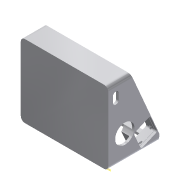
# Autodesk Inventor part: 03_OpenOxygen_Box
Saved by Autodesk Inventor 2019.4 (Build 234330000, 330)
## iProperties
Created: 2021-06-03
Part Number: 03_OpenOxygen_Box
Material: Generic
Document SubType Name: Modeling
Designer: diederichbenedict
Density: 1 g/cm^3
Appearance: Snow
Author: diederichbenedict
Autodesk Inventor part; units mm, degrees
(part 1 of 2)
ref_plane "YZ Plane" through (0, 0, 0) normal (1, 0, 0) x (0, 1, 0)
ref_plane "XZ Plane" through (0, 0, 0) normal (0, 1, 0) x (-1, 0, 0)
ref_plane "Work Plane1" through (0, 0, 0) normal (0, 0, 1) x (1, 0, 0)
sketch "Sketch1" plane through (0, 0, 0) normal (0, 0, 1) x (1, 0, 0)
  line L0 (30.9254, 0.1) -> (30.9254, 0) projected
  line L1 (30.9254, 0) -> (32.2546, 0) projected
  line L2 (32.2546, 0) -> (32.2546, 0.1) projected
  line L3 (32.2546, 0.1) -> (33.4654, 0.1) projected
  line L4 (33.4654, 0.1) -> (33.4654, 0) projected
  line L5 (33.4654, 0) -> (34.7946, 0) projected
  line L6 (34.7946, 0) -> (34.7946, 0.1) projected
  line L7 (34.7946, 0.1) -> (36.0054, 0.1) projected
  line L8 (36.0054, 0.1) -> (36.0054, 0) projected
  line L9 (36.0054, 0) -> (37.3346, 0) projected
  line L10 (37.3346, 0) -> (37.3346, 0.1) projected
  line L11 (37.3346, 0.1) -> (38.5454, 0.1) projected
  line L12 (38.5454, 0.1) -> (38.5454, 0) projected
  line L13 (38.5454, 0) -> (39.8746, 0) projected
  line L14 (39.8746, 0) -> (39.8746, 0.1) projected
  line L15 (39.8746, 0.1) -> (41.0854, 0.1) projected
  line L16 (41.0854, 0.1) -> (41.0854, 0) projected
  line L17 (41.0854, 0) -> (42.4146, 0) projected
  line L18 (42.4146, 0) -> (42.4146, 0.1) projected
  line L19 (42.4146, 0.1) -> (43.6254, 0.1) projected
  line L20 (43.6254, 0.1) -> (43.6254, 0) projected
  line L21 (43.6254, 0) -> (44.9546, 0) projected
  line L22 (44.9546, 0) -> (44.9546, 0.1) projected
  line L23 (44.9546, 0.1) -> (46.1654, 0.1) projected
  line L24 (46.1654, 0.1) -> (46.1654, 0) projected
  line L25 (46.1654, 0) -> (47.4946, 0) projected
  line L26 (47.4946, 0) -> (47.4946, 0.1) projected
  line L27 (47.4946, 0.1) -> (48.7054, 0.1) projected
  line L28 (48.7054, 0.1) -> (48.7054, 0) projected
  line L29 (48.7054, 0) -> (98, 0) projected
  line L30 (98, 0) -> (98, 1.6) projected
  line L31 (0, 1.6) -> (98, 1.6) projected
  line L32 (0, 0) -> (0, 1.6) projected
  line L33 (0, 0) -> (9.3946, 0) projected
  line L34 (9.3946, 0) -> (9.3946, 0.1) projected
  line L35 (9.3946, 0.1) -> (10.6054, 0.1) projected
  line L36 (10.6054, 0.1) -> (10.6054, 0) projected
  line L37 (10.6054, 0) -> (11.9346, 0) projected
  line L38 (11.9346, 0) -> (11.9346, 0.1) projected
  line L39 (11.9346, 0.1) -> (13.1454, 0.1) projected
  line L40 (13.1454, 0.1) -> (13.1454, 0) projected
  line L41 (13.1454, 0) -> (14.4746, 0) projected
  line L42 (14.4746, 0) -> (14.4746, 0.1) projected
  line L43 (14.4746, 0.1) -> (15.6854, 0.1) projected
  line L44 (15.6854, 0.1) -> (15.6854, 0) projected
  line L45 (15.6854, 0) -> (17.0146, 0) projected
  line L46 (17.0146, 0) -> (17.0146, 0.1) projected
  line L47 (17.0146, 0.1) -> (18.2254, 0.1) projected
  line L48 (18.2254, 0.1) -> (18.2254, 0) projected
  line L49 (18.2254, 0) -> (19.5546, 0) projected
  line L50 (19.5546, 0) -> (19.5546, 0.1) projected
  line L51 (19.5546, 0.1) -> (20.7654, 0.1) projected
  line L52 (20.7654, 0.1) -> (20.7654, 0) projected
  line L53 (20.7654, 0) -> (22.0946, 0) projected
  line L54 (22.0946, 0) -> (22.0946, 0.1) projected
  line L55 (22.0946, 0.1) -> (23.3054, 0.1) projected
  line L56 (23.3054, 0.1) -> (23.3054, 0) projected
  line L57 (23.3054, 0) -> (24.6346, 0) projected
  line L58 (24.6346, 0) -> (24.6346, 0.1) projected
  line L59 (24.6346, 0.1) -> (25.8454, 0.1) projected
  line L60 (25.8454, 0.1) -> (25.8454, 0) projected
  line L61 (25.8454, 0) -> (27.1746, 0) projected
  line L62 (27.1746, 0) -> (27.1746, 0.1) projected
  line L63 (27.1746, 0.1) -> (28.3854, 0.1) projected
  line L64 (28.3854, 0.1) -> (28.3854, 0) projected
  line L65 (28.3854, 0) -> (29.7146, 0) projected
  line L66 (29.7146, 0) -> (29.7146, 0.1) projected
  line L67 (29.7146, 0.1) -> (30.9254, 0.1) projected
  line L68 (63.1351, 91.3523) -> (63.1351, 51.3523) projected
  line L69 (49.1351, 91.3523) -> (63.1351, 91.3523) projected
  line L70 (49.1351, 51.3523) -> (49.1351, 91.3523) projected
  line L71 (63.1351, 51.3523) -> (49.1351, 51.3523) projected
  line L72 (0, 1.6) -> (98, 1.6)
  line L73 (103, 6.6) -> (103, 86.6)
  line L74 (98, 91.6) -> (0, 91.6)
  line L75 (-5, 86.6) -> (-5, 6.6)
  arc A0 (98, 1.6) -> (103, 6.6) centre (98, 6.6) ccw
  arc A1 (103, 86.6) -> (98, 91.6) centre (98, 86.6) ccw
  arc A2 (0, 91.6) -> (-5, 86.6) centre (0, 86.6) ccw
  arc A3 (-5, 6.6) -> (0, 1.6) centre (0, 6.6) ccw
  point P0 (-5, 1.6)
  point P1 (103, 91.6)
  point P2 (103, 1.6)
  point P3 (-5, 91.6)
  dimension "d1" = 5
  dimension "d2" = 5
  dimension "d3" = 90
  dimension "d6" = 5
  constraints: 9 point on line, 8 end point, 8 point on circle, 8 tangent, 4 centre point, 3 equal radius, 2 parallel, 1 horizontal, 1 perpendicular
  measures "d1" distance between parallel lines of L32 L75
  measures "d2" distance between parallel lines of L30 L73
  measures "d3" distance between parallel lines of L72 L74
  measures "d6" radius of A0
extrude "Extrusion1" add sketch "Sketch1" along normal blind 3 contours L31 A3 L75 A2 L74 A1 L73 A0 | L68 L71 L70 L69
sketch "Sketch2" plane through (0, 0, 0) normal (0, 0, -1) x (-1, 0, 0)
  arc A0 (0, 1.6) -> (5, 6.6) centre (0, 6.6) ccw projected
  line L0 (5, 6.6) -> (5, 86.6) projected
  arc A1 (5, 86.6) -> (0, 91.6) centre (0, 86.6) ccw projected
  line L1 (0, 91.6) -> (-98, 91.6) projected
  arc A2 (-98, 91.6) -> (-103, 86.6) centre (-98, 86.6) ccw projected
  line L2 (-103, 86.6) -> (-103, 6.6) projected
  arc A3 (-103, 6.6) -> (-98, 1.6) centre (-98, 6.6) ccw projected
  line L3 (-98, 1.6) -> (0, 1.6) projected
  line L4 (-100, 6.6) -> (-100, 86.6)
  arc A4 (-98, 88.6) -> (-100, 86.6) centre (-98, 86.6) ccw
  line L5 (-98, 88.6) -> (0, 88.6)
  arc A5 (2, 86.6) -> (0, 88.6) centre (0, 86.6) ccw
  line L6 (2, 86.6) -> (2, 6.6)
  arc A6 (0, 4.6) -> (2, 6.6) centre (0, 6.6) ccw
  line L7 (0, 4.6) -> (-98, 4.6)
  arc A7 (-100, 6.6) -> (-98, 4.6) centre (-98, 6.6) ccw
  point P0 (0, 0)
  dimension "d7" = 3
  constraints: 8 end point, 8 point on circle, 4 centre point, 7 other
  measures "d7" distance between parallel lines of L2 L4
ref_plane "Work Plane2" through (0, 0, -60) normal (0, 0, -1) x (0, 1, 0)
extrude "Extrusion2" add sketch "Sketch2" along normal up to surface (60 mm away)
sketch "Sketch3" plane through (-5, 6.6, 3) normal (-1, 0, 0) x (0, 0, 1)
  line L0 (0, 0) -> (-63, 0) projected
  line L1 (0, 80) -> (0, 0) projected
  line L2 (0, 80) -> (-63, 80) projected
  line L3 (-63, 80) -> (-63, 0) projected
  line L4 (-63, 4.0286) -> (-27.0673, 87.1327)
  line L5 (-27.0673, 87.1327) -> (-72.7137, 86.3795)
  line L6 (-72.7137, 86.3795) -> (-69.4498, 6.2882)
  line L7 (-69.4498, 6.2882) -> (-63, 4.0286)
  point P0 (-3, -6.6)
  constraints: 8 end point, 1 point on line
extrude "Extrusion3" cut sketch "Sketch3" against normal through all contours L7 L6 L5 L4 L2 L3 | L3 L2 L4
sketch "Sketch4" plane through (-5, 6.6, 3) normal (-1, 0, 0) x (0, 0, 1)
  circle A0 centre (-20.557, 24.8509) radius 11.8979 projected
  point P0 (-3, -6.6)
extrude "Extrusion4" cut sketch "Sketch4" against normal through all
sketch "Sketch5" plane through (0, 1.6, 3) normal (0, -1, 0) x (1, 0, 0)
  circle A0 centre (95.5, -5.5) radius 1.5 projected
  circle A1 centre (95.5, -60.5) radius 1.5 projected
  circle A2 centre (2.5, -60.5) radius 1.5 projected
  circle A3 centre (2.5, -5.5) radius 1.5 projected
  line L0 (8.1, -22.25) -> (8.1, -4.25) construction
  line L1 (8.1, -4.25) -> (49.6, -4.25) construction
  line L2 (49.6, -4.25) -> (49.6, -22.25) construction
  line L3 (49.6, -22.25) -> (8.1, -22.25) construction
  circle A4 centre (43.02, -5.5) radius 0.75 construction
  circle A5 centre (40.48, -5.5) radius 0.75 construction
  circle A6 centre (37.94, -5.5) radius 0.75 construction
  circle A7 centre (35.4, -5.5) radius 0.75 construction
  circle A8 centre (32.86, -5.5) radius 0.75 construction
  circle A9 centre (30.32, -5.5) radius 0.75 construction
  circle A10 centre (27.78, -5.5) radius 0.75 construction
  circle A11 centre (25.24, -5.5) radius 0.75 construction
  circle A12 centre (22.7, -5.5) radius 0.75 construction
  circle A13 centre (20.16, -5.5) radius 0.75 construction
  circle A14 centre (17.62, -5.5) radius 0.75 construction
  circle A15 centre (15.08, -5.5) radius 0.75 construction
  circle A16 centre (12.54, -5.5) radius 0.75 construction
  circle A17 centre (10, -5.5) radius 0.75 construction
  line L4 (21.6, -15.05) -> (14.6, -15.05) construction
  line L5 (21.6, -8.05) -> (21.6, -15.05) construction
  line L6 (14.6, -8.05) -> (21.6, -8.05) construction
  line L7 (14.6, -15.05) -> (14.6, -8.05) construction
  line L8 (20.85, -20.75) -> (19.85, -20.75) construction
  line L9 (20.85, -19.25) -> (20.85, -20.75) construction
  line L10 (19.85, -19.25) -> (20.85, -19.25) construction
  line L11 (19.85, -20.75) -> (19.85, -19.25) construction
  line L12 (20.85, -18.75) -> (19.85, -18.75) construction
  line L13 (20.85, -17.25) -> (20.85, -18.75) construction
  line L14 (19.85, -17.25) -> (20.85, -17.25) construction
  line L15 (19.85, -18.75) -> (19.85, -17.25) construction
  line L16 (17.85, -20.75) -> (17.85, -19.25) construction
  line L17 (18.85, -20.75) -> (17.85, -20.75) construction
  line L18 (18.85, -19.25) -> (18.85, -20.75) construction
  line L19 (17.85, -19.25) -> (18.85, -19.25) construction
  line L20 (17.85, -18.75) -> (17.85, -17.25) construction
  line L21 (18.85, -18.75) -> (17.85, -18.75) construction
  line L22 (18.85, -17.25) -> (18.85, -18.75) construction
  line L23 (17.85, -17.25) -> (18.85, -17.25) construction
  line L24 (15.85, -20.75) -> (15.85, -19.25) construction
  line L25 (16.85, -20.75) -> (15.85, -20.75) construction
  line L26 (16.85, -19.25) -> (16.85, -20.75) construction
  line L27 (15.85, -19.25) -> (16.85, -19.25) construction
  line L28 (15.85, -18.75) -> (15.85, -17.25) construction
  line L29 (16.85, -18.75) -> (15.85, -18.75) construction
  line L30 (16.85, -17.25) -> (16.85, -18.75) construction
  line L31 (15.85, -17.25) -> (16.85, -17.25) construction
  line L32 (36.6, -19.725) -> (37.6, -19.725) construction
  line L33 (36.6, -19.75) -> (36.6, -19.725) construction
  line L34 (36.1, -19.75) -> (36.6, -19.75) construction
  line L35 (36.1, -21) -> (36.1, -19.75) construction
  line L36 (36.6, -21) -> (36.1, -21) construction
  line L37 (36.6, -21.025) -> (36.6, -21) construction
  line L38 (37.6, -21.025) -> (36.6, -21.025) construction
  line L39 (37.6, -21) -> (37.6, -21.025) construction
  line L40 (38.1, -21) -> (37.6, -21) construction
  line L41 (38.1, -19.75) -> (38.1, -21) construction
  line L42 (37.6, -19.75) -> (38.1, -19.75) construction
  line L43 (37.6, -19.725) -> (37.6, -19.75) construction
  line L44 (31.6, -21) -> (31.1, -21) construction
  line L45 (31.6, -21.025) -> (31.6, -21) construction
  line L46 (32.6, -21.025) -> (31.6, -21.025) construction
  line L47 (32.6, -21) -> (32.6, -21.025) construction
  line L48 (33.1, -21) -> (32.6, -21) construction
  line L49 (33.1, -19.75) -> (33.1, -21) construction
  line L50 (32.6, -19.75) -> (33.1, -19.75) construction
  line L51 (32.6, -19.725) -> (32.6, -19.75) construction
  line L52 (31.6, -19.725) -> (32.6, -19.725) construction
  line L53 (31.6, -19.75) -> (31.6, -19.725) construction
  line L54 (31.1, -19.75) -> (31.6, -19.75) construction
  line L55 (31.1, -21) -> (31.1, -19.75) construction
  line L56 (26.6, -21) -> (26.1, -21) construction
  line L57 (26.6, -21.025) -> (26.6, -21) construction
  line L58 (27.6, -21.025) -> (26.6, -21.025) construction
  line L59 (27.6, -21) -> (27.6, -21.025) construction
  line L60 (28.1, -21) -> (27.6, -21) construction
  line L61 (28.1, -19.75) -> (28.1, -21) construction
  line L62 (27.6, -19.75) -> (28.1, -19.75) construction
  line L63 (27.6, -19.725) -> (27.6, -19.75) construction
  line L64 (26.6, -19.725) -> (27.6, -19.725) construction
  line L65 (26.6, -19.75) -> (26.6, -19.725) construction
  line L66 (26.1, -19.75) -> (26.6, -19.75) construction
  line L67 (26.1, -21) -> (26.1, -19.75) construction
  line L68 (45.1607, -15.4113) -> (45.1607, -14.9113) construction
  line L69 (45.1357, -15.4113) -> (45.1607, -15.4113) construction
  line L70 (45.1357, -16.4113) -> (45.1357, -15.4113) construction
  line L71 (45.1607, -16.4113) -> (45.1357, -16.4113) construction
  line L72 (45.1607, -16.9113) -> (45.1607, -16.4113) construction
  line L73 (46.4107, -16.9113) -> (45.1607, -16.9113) construction
  line L74 (46.4107, -16.4113) -> (46.4107, -16.9113) construction
  line L75 (46.4357, -16.4113) -> (46.4107, -16.4113) construction
  line L76 (46.4357, -15.4113) -> (46.4357, -16.4113) construction
  line L77 (46.4107, -15.4113) -> (46.4357, -15.4113) construction
  line L78 (46.4107, -14.9113) -> (46.4107, -15.4113) construction
  line L79 (45.1607, -14.9113) -> (46.4107, -14.9113) construction
  line L80 (42.6357, -16.4113) -> (42.6357, -15.4113) construction
  line L81 (42.6607, -16.4113) -> (42.6357, -16.4113) construction
  line L82 (42.6607, -16.9113) -> (42.6607, -16.4113) construction
  line L83 (43.9107, -16.9113) -> (42.6607, -16.9113) construction
  line L84 (43.9107, -16.4113) -> (43.9107, -16.9113) construction
  line L85 (43.9357, -16.4113) -> (43.9107, -16.4113) construction
  line L86 (43.9357, -15.4113) -> (43.9357, -16.4113) construction
  line L87 (43.9107, -15.4113) -> (43.9357, -15.4113) construction
  line L88 (43.9107, -14.9113) -> (43.9107, -15.4113) construction
  line L89 (42.6607, -14.9113) -> (43.9107, -14.9113) construction
  line L90 (42.6607, -15.4113) -> (42.6607, -14.9113) construction
  line L91 (42.6357, -15.4113) -> (42.6607, -15.4113) construction
  line L92 (40.1357, -16.4113) -> (40.1357, -15.4113) construction
  line L93 (40.1607, -16.4113) -> (40.1357, -16.4113) construction
  line L94 (40.1607, -16.9113) -> (40.1607, -16.4113) construction
  line L95 (41.4107, -16.9113) -> (40.1607, -16.9113) construction
  line L96 (41.4107, -16.4113) -> (41.4107, -16.9113) construction
  line L97 (41.4357, -16.4113) -> (41.4107, -16.4113) construction
  line L98 (41.4357, -15.4113) -> (41.4357, -16.4113) construction
  line L99 (41.4107, -15.4113) -> (41.4357, -15.4113) construction
  line L100 (41.4107, -14.9113) -> (41.4107, -15.4113) construction
  line L101 (40.1607, -14.9113) -> (41.4107, -14.9113) construction
  line L102 (40.1607, -15.4113) -> (40.1607, -14.9113) construction
  line L103 (40.1357, -15.4113) -> (40.1607, -15.4113) construction
  line L104 (37.6357, -16.4113) -> (37.6357, -15.4113) construction
  line L105 (37.6607, -16.4113) -> (37.6357, -16.4113) construction
  line L106 (37.6607, -16.9113) -> (37.6607, -16.4113) construction
  line L107 (38.9107, -16.9113) -> (37.6607, -16.9113) construction
  line L108 (38.9107, -16.4113) -> (38.9107, -16.9113) construction
  line L109 (38.9357, -16.4113) -> (38.9107, -16.4113) construction
  line L110 (38.9357, -15.4113) -> (38.9357, -16.4113) construction
  line L111 (38.9107, -15.4113) -> (38.9357, -15.4113) construction
  line L112 (38.9107, -14.9113) -> (38.9107, -15.4113) construction
  line L113 (37.6607, -14.9113) -> (38.9107, -14.9113) construction
  line L114 (37.6607, -15.4113) -> (37.6607, -14.9113) construction
  line L115 (37.6357, -15.4113) -> (37.6607, -15.4113) construction
  line L116 (40.1607, -10.9113) -> (40.1607, -10.4113) construction
  line L117 (40.1357, -10.9113) -> (40.1607, -10.9113) construction
  line L118 (40.1357, -11.9113) -> (40.1357, -10.9113) construction
  line L119 (40.1607, -11.9113) -> (40.1357, -11.9113) construction
  line L120 (40.1607, -12.4113) -> (40.1607, -11.9113) construction
  line L121 (41.4107, -12.4113) -> (40.1607, -12.4113) construction
  line L122 (41.4107, -11.9113) -> (41.4107, -12.4113) construction
  line L123 (41.4357, -11.9113) -> (41.4107, -11.9113) construction
  line L124 (41.4357, -10.9113) -> (41.4357, -11.9113) construction
  line L125 (41.4107, -10.9113) -> (41.4357, -10.9113) construction
  line L126 (41.4107, -10.4113) -> (41.4107, -10.9113) construction
  line L127 (40.1607, -10.4113) -> (41.4107, -10.4113) construction
  line L128 (37.6357, -11.9113) -> (37.6357, -10.9113) construction
  line L129 (37.6607, -11.9113) -> (37.6357, -11.9113) construction
  line L130 (37.6607, -12.4113) -> (37.6607, -11.9113) construction
  line L131 (38.9107, -12.4113) -> (37.6607, -12.4113) construction
  line L132 (38.9107, -11.9113) -> (38.9107, -12.4113) construction
  line L133 (38.9357, -11.9113) -> (38.9107, -11.9113) construction
  line L134 (38.9357, -10.9113) -> (38.9357, -11.9113) construction
  line L135 (38.9107, -10.9113) -> (38.9357, -10.9113) construction
  line L136 (38.9107, -10.4113) -> (38.9107, -10.9113) construction
  line L137 (37.6607, -10.4113) -> (38.9107, -10.4113) construction
  line L138 (37.6607, -10.9113) -> (37.6607, -10.4113) construction
  line L139 (37.6357, -10.9113) -> (37.6607, -10.9113) construction
  line L140 (43.4, -11.75) -> (43.2, -11.75) construction
  line L141 (43.4, -12.45) -> (43.4, -11.75) construction
  line L142 (43.9, -12.45) -> (43.4, -12.45) construction
  line L143 (43.9, -11.75) -> (43.9, -12.45) construction
  line L144 (45.2, -11.75) -> (43.9, -11.75) construction
  line L145 (45.2, -12.45) -> (45.2, -11.75) construction
  line L146 (45.7, -12.45) -> (45.2, -12.45) construction
  line L147 (45.7, -11.75) -> (45.7, -12.45) construction
  line L148 (45.9, -11.75) -> (45.7, -11.75) construction
  line L149 (45.9, -10.25) -> (45.9, -11.75) construction
  line L150 (44.8, -10.25) -> (45.9, -10.25) construction
  line L151 (44.8, -9.55) -> (44.8, -10.25) construction
  line L152 (44.3, -9.55) -> (44.8, -9.55) construction
  line L153 (44.3, -10.25) -> (44.3, -9.55) construction
  line L154 (43.2, -10.25) -> (44.3, -10.25) construction
  line L155 (43.2, -11.75) -> (43.2, -10.25) construction
  line L156 (11.6965, -17.6363) -> (11.6965, -16.6863) construction
  line L157 (11.6965, -16.6863) -> (11.6112, -16.6863) construction
  line L158 (11.6112, -16.6863) -> (11.6112, -17.5389) construction
  line L159 (11.6112, -17.5389) -> (11.2458, -17.5389) construction
  line L160 (11.2458, -17.5389) -> (11.2458, -17.6363) construction
  line L161 (11.2458, -17.6363) -> (11.6965, -17.6363) construction
  spline S0 degree 3 poles (12.3058, -16.662) (12.2949, -16.6621) (12.2733, -16.6624) (12.2413, -16.6649) (12.2102, -16.6691) (12.1799, -16.6748) (12.1503, -16.6819) (12.1216, -16.6912) (12.0936, -16.7018) (12.0665, -16.714) (12.0405, -16.7277) (12.0155, -16.7427) (11.9918, -16.7591) (11.9691, -16.7767) (11.9479, -16.7958) (11.9276, -16.8159) (11.9088, -16.8377) (11.8972, -16.853) (11.8913, -16.8607) knots 0 0 0 0 0.068548 0.135683 0.201215 0.265682 0.329267 0.392395 0.45507 0.517127 0.57879 0.63974 0.700192 0.759806 0.819628 0.879355 0.939512 1 1 1 1 construction
  line L162 (11.8913, -16.8607) -> (11.9659, -16.9177) construction
  spline S1 degree 3 poles (11.9659, -16.9177) (11.9713, -16.9114) (11.9818, -16.8988) (11.9988, -16.8811) (12.0166, -16.8645) (12.035, -16.849) (12.0545, -16.835) (12.0745, -16.8219) (12.0955, -16.8102) (12.1245, -16.796) (12.1624, -16.7811) (12.2101, -16.7686) (12.2599, -16.7607) (12.2939, -16.7598) (12.3112, -16.7594) knots 0 0 0 0 0.063163 0.125475 0.187121 0.248294 0.309295 0.36985 0.430973 0.492456 0.616148 0.740844 0.868183 1 1 1 1 construction
  spline S2 degree 3 poles (12.3112, -16.7594) (12.3207, -16.7595) (12.3396, -16.7597) (12.3678, -16.7626) (12.3954, -16.7667) (12.4224, -16.7727) (12.4489, -16.7803) (12.475, -16.7893) (12.5003, -16.8006) (12.5252, -16.813) (12.549, -16.827) (12.5716, -16.8423) (12.5927, -16.8587) (12.6126, -16.8762) (12.6311, -16.8948) (12.6481, -16.9147) (12.6636, -16.9359) (12.6779, -16.9579) (12.6908, -16.9809) (12.7015, -17.0048) (12.711, -17.0293) (12.7185, -17.0545) (12.7245, -17.0805) (12.7286, -17.1071) (12.7314, -17.1344) (12.7316, -17.153) (12.7317, -17.1623) knots 0 0 0 0 0.043955 0.087502 0.130463 0.172752 0.215403 0.25765 0.300153 0.343121 0.385925 0.427686 0.468818 0.509492 0.549883 0.58998 0.630405 0.670869 0.711384 0.751627 0.791776 0.832459 0.873319 0.914543 0.956924 1 1 1 1 construction
  spline S3 degree 3 poles (12.7317, -17.1623) (12.7314, -17.1763) (12.7307, -17.2039) (12.7247, -17.2443) (12.7156, -17.283) (12.702, -17.3197) (12.6852, -17.355) (12.664, -17.3881) (12.6394, -17.4197) (12.6111, -17.449) (12.58, -17.4758) (12.5467, -17.4993) (12.5112, -17.5189) (12.4739, -17.5353) (12.4345, -17.5478) (12.3932, -17.5567) (12.3499, -17.5624) (12.3203, -17.563) (12.3053, -17.5633) knots 0 0 0 0 0.064323 0.12629 0.186726 0.246146 0.305576 0.365429 0.426326 0.48884 0.551725 0.613919 0.675484 0.737334 0.800229 0.864502 0.931041 1 1 1 1 construction
  spline S4 degree 3 poles (12.3053, -17.5633) (12.2887, -17.5628) (12.256, -17.5619) (12.2082, -17.5543) (12.1623, -17.5419) (12.1186, -17.5245) (12.0769, -17.502) (12.0374, -17.4746) (12, -17.4423) (11.9774, -17.4175) (11.9659, -17.4049) knots 0 0 0 0 0.128515 0.252949 0.374755 0.49594 0.617181 0.740909 0.867811 1 1 1 1 construction
  line L163 (11.9659, -17.4049) -> (11.8913, -17.4614) construction
  spline S5 degree 3 poles (11.8913, -17.4614) (11.8974, -17.4692) (11.9093, -17.4846) (11.9287, -17.5064) (11.9492, -17.5269) (11.9708, -17.546) (11.9933, -17.5639) (12.0172, -17.5803) (12.0422, -17.5953) (12.0681, -17.609) (12.0949, -17.6212) (12.1226, -17.6317) (12.151, -17.6407) (12.1802, -17.6481) (12.2103, -17.6538) (12.2411, -17.6577) (12.2726, -17.6603) (12.2939, -17.6606) (12.3047, -17.6607) knots 0 0 0 0 0.061674 0.123053 0.183475 0.243727 0.304279 0.364863 0.425946 0.487391 0.54922 0.611144 0.673529 0.736961 0.800785 0.866013 0.932101 1 1 1 1 construction
  spline S6 degree 3 poles (12.3047, -17.6607) (12.3149, -17.6606) (12.3351, -17.6605) (12.3649, -17.6582) (12.394, -17.6551) (12.4221, -17.6504) (12.4496, -17.6449) (12.4761, -17.6375) (12.5019, -17.6292) (12.5268, -17.6195) (12.551, -17.6085) (12.5743, -17.596) (12.5967, -17.5823) (12.6185, -17.5675) (12.6393, -17.5512) (12.6593, -17.5337) (12.6786, -17.5149) (12.6905, -17.5014) (12.6965, -17.4946) knots 0 0 0 0 0.069663 0.13775 0.203917 0.26878 0.332414 0.394754 0.45618 0.516996 0.577396 0.637198 0.696999 0.756756 0.816554 0.876948 0.938132 1 1 1 1 construction
  spline S7 degree 3 poles (12.6965, -17.4946) (12.7061, -17.4827) (12.7253, -17.4592) (12.7497, -17.4212) (12.7707, -17.3814) (12.7876, -17.3398) (12.8008, -17.2963) (12.81, -17.2511) (12.816, -17.2041) (12.8166, -17.1721) (12.817, -17.1558) knots 0 0 0 0 0.124329 0.247156 0.36878 0.490734 0.613614 0.738958 0.867311 1 1 1 1 construction
  spline S8 degree 3 poles (12.817, -17.1558) (12.8166, -17.1387) (12.8157, -17.1051) (12.8087, -17.0558) (12.7973, -17.0085) (12.7812, -16.9634) (12.7608, -16.9202) (12.7355, -16.8793) (12.7058, -16.8403) (12.6717, -16.8039) (12.6344, -16.7707) (12.5944, -16.7414) (12.5518, -16.717) (12.5072, -16.6967) (12.4601, -16.681) (12.4107, -16.6701) (12.359, -16.6633) (12.3237, -16.6624) (12.3058, -16.662) knots 0 0 0 0 0.064558 0.127014 0.187955 0.248014 0.307748 0.368235 0.42947 0.492743 0.556258 0.618217 0.679655 0.741246 0.803415 0.866815 0.932328 1 1 1 1 construction
  spline S9 degree 3 poles (13.2345, -17.6607) (13.2417, -17.6606) (13.256, -17.6603) (13.277, -17.6578) (13.2977, -17.6544) (13.3177, -17.6489) (13.3372, -17.6423) (13.3563, -17.6341) (13.3748, -17.6243) (13.393, -17.6131) (13.4106, -17.6) (13.4277, -17.5848) (13.4448, -17.5679) (13.4612, -17.5488) (13.4775, -17.5278) (13.4932, -17.5047) (13.5087, -17.4797) (13.5184, -17.4621) (13.5234, -17.4531) knots 0 0 0 0 0.057208 0.113696 0.169178 0.224159 0.27872 0.333794 0.389241 0.445822 0.503704 0.564294 0.627975 0.695038 0.765373 0.839611 0.917538 1 1 1 1 construction
  line L164 (13.5234, -17.4531) -> (13.4431, -17.4049) construction
  spline S10 degree 3 poles (13.4431, -17.4049) (13.4356, -17.4174) (13.4213, -17.4414) (13.3974, -17.4738) (13.3727, -17.5013) (13.3469, -17.5238) (13.3202, -17.5415) (13.2925, -17.554) (13.2638, -17.5618) (13.2443, -17.5628) (13.2345, -17.5633) knots 0 0 0 0 0.159004 0.304646 0.438547 0.562322 0.677433 0.786897 0.893611 1 1 1 1 construction
  spline S11 degree 3 poles (13.2345, -17.5633) (13.2262, -17.563) (13.2097, -17.5626) (13.1854, -17.5581) (13.1618, -17.5514) (13.1393, -17.5416) (13.1184, -17.5299) (13.1001, -17.5157) (13.0842, -17.4998) (13.0712, -17.482) (13.0613, -17.4629) (13.0536, -17.4433) (13.0494, -17.4229) (13.0487, -17.4092) (13.0484, -17.4023) knots 0 0 0 0 0.091264 0.18093 0.270088 0.360156 0.448343 0.532666 0.613834 0.693982 0.772716 0.849335 0.923967 1 1 1 1 construction
  spline S12 degree 3 poles (13.0484, -17.4023) (13.0488, -17.3943) (13.0496, -17.3783) (13.0565, -17.3545) (13.0673, -17.3311) (13.0773, -17.3165) (13.0825, -17.309) knots 0 0 0 0 0.234723 0.477158 0.728556 1 1 1 1 construction
  spline S13 degree 3 poles (13.0825, -17.309) (13.0867, -17.3036) (13.0956, -17.2921) (13.111, -17.2751) (13.129, -17.2576) (13.1491, -17.2389) (13.1719, -17.2198) (13.1968, -17.1995) (13.2244, -17.1787) (13.2438, -17.1647) (13.2537, -17.1575) knots 0 0 0 0 0.090279 0.18953 0.299198 0.418926 0.548376 0.688136 0.839084 1 1 1 1 construction
  spline S14 degree 3 poles (13.2537, -17.1575) (13.2637, -17.1504) (13.2828, -17.1368) (13.3096, -17.1166) (13.3335, -17.0981) (13.3544, -17.0812) (13.3725, -17.0659) (13.3877, -17.0522) (13.3997, -17.0399) (13.4064, -17.0319) (13.4094, -17.0283) knots 0 0 0 0 0.181535 0.347082 0.495568 0.628357 0.74552 0.845831 0.930782 1 1 1 1 construction
  spline S15 degree 3 poles (13.4094, -17.0283) (13.4136, -17.0227) (13.4219, -17.0117) (13.4328, -16.9945) (13.442, -16.9769) (13.4493, -16.9589) (13.4554, -16.9406) (13.4595, -16.922) (13.4621, -16.9029) (13.4624, -16.8901) (13.4625, -16.8837) knots 0 0 0 0 0.133507 0.262559 0.388264 0.512667 0.633722 0.755394 0.877553 1 1 1 1 construction
  spline S16 degree 3 poles (13.4625, -16.8837) (13.4621, -16.8736) (13.4614, -16.8537) (13.4555, -16.8247) (13.4462, -16.797) (13.4331, -16.7708) (13.4162, -16.7469) (13.3966, -16.725) (13.3733, -16.7067) (13.3478, -16.6906) (13.3198, -16.678) (13.2905, -16.6685) (13.2598, -16.6631) (13.239, -16.6624) (13.2284, -16.662) knots 0 0 0 0 0.083785 0.16578 0.24628 0.327461 0.408797 0.489715 0.571376 0.655523 0.741019 0.826547 0.911989 1 1 1 1 construction
  spline S17 degree 3 poles (13.2284, -16.662) (13.2172, -16.6624) (13.195, -16.6631) (13.1622, -16.6698) (13.1307, -16.6809) (13.1053, -16.6934) (13.0855, -16.7059) (13.0703, -16.7173) (13.055, -16.7304) (13.0393, -16.7453) (13.0236, -16.7621) (13.0076, -16.7807) (12.9912, -16.8009) (12.9807, -16.8154) (12.9753, -16.8228) knots 0 0 0 0 0.107233 0.213252 0.31883 0.426794 0.483646 0.543604 0.608308 0.677127 0.750686 0.828713 0.91219 1 1 1 1 construction
  line L165 (12.9753, -16.8228) -> (13.0524, -16.8812) construction
  spline S18 degree 3 poles (13.0524, -16.8812) (13.0571, -16.8752) (13.066, -16.8637) (13.0796, -16.8475) (13.0924, -16.8327) (13.1051, -16.8199) (13.1169, -16.8083) (13.1283, -16.7984) (13.1392, -16.79) (13.153, -16.7811) (13.1703, -16.7723) (13.192, -16.7648) (13.2147, -16.7603) (13.2301, -16.7597) (13.2379, -16.7594) knots 0 0 0 0 0.098469 0.189629 0.274184 0.352183 0.423199 0.488551 0.548473 0.60144 0.701198 0.799592 0.898545 1 1 1 1 construction
  spline S19 degree 3 poles (13.2379, -16.7594) (13.2478, -16.7597) (13.2667, -16.7604) (13.2936, -16.7673) (13.3177, -16.7782) (13.3385, -16.7935) (13.3558, -16.8116) (13.3683, -16.8324) (13.3759, -16.8555) (13.3768, -16.8715) (13.3772, -16.8797) knots 0 0 0 0 0.143073 0.275903 0.402371 0.528414 0.650356 0.765895 0.880774 1 1 1 1 construction
  spline S20 degree 3 poles (13.3772, -16.8797) (13.3771, -16.8848) (13.3769, -16.895) (13.3739, -16.91) (13.3701, -16.925) (13.3641, -16.9399) (13.3557, -16.955) (13.3447, -16.9705) (13.3308, -16.9865) (13.3202, -16.9969) (13.3146, -17.0024) knots 0 0 0 0 0.107285 0.214746 0.322939 0.434116 0.553412 0.686073 0.834256 1 1 1 1 construction
  spline S21 degree 3 poles (13.3146, -17.0024) (13.3126, -17.0043) (13.3076, -17.0087) (13.2986, -17.0159) (13.2867, -17.0248) (13.2721, -17.0358) (13.2548, -17.0486) (13.2346, -17.063) (13.2117, -17.0794) (13.1955, -17.0909) (13.1869, -17.097) knots 0 0 0 0 0.052594 0.124952 0.218094 0.333502 0.468789 0.624938 0.801683 1 1 1 1 construction
  spline S22 degree 3 poles (13.1869, -17.097) (13.1766, -17.1045) (13.1567, -17.119) (13.1283, -17.1409) (13.1025, -17.1622) (13.0793, -17.1829) (13.0584, -17.2029) (13.0401, -17.2223) (13.0242, -17.2411) (13.0071, -17.2651) (12.9895, -17.2946) (12.9745, -17.3308) (12.965, -17.3671) (12.9638, -17.3915) (12.9631, -17.4036) knots 0 0 0 0 0.096972 0.187773 0.272396 0.351321 0.424335 0.491909 0.554233 0.611268 0.716348 0.81454 0.908495 1 1 1 1 construction
  spline S23 degree 3 poles (12.9631, -17.4036) (12.9633, -17.4121) (12.9637, -17.429) (12.9677, -17.4537) (12.9737, -17.4778) (12.9827, -17.5008) (12.9936, -17.5233) (13.0075, -17.5446) (13.0236, -17.5652) (13.0421, -17.5845) (13.0623, -17.6022) (13.0836, -17.618) (13.1062, -17.6312) (13.1298, -17.6419) (13.1544, -17.6503) (13.1802, -17.6564) (13.207, -17.6601) (13.2252, -17.6605) (13.2345, -17.6607) knots 0 0 0 0 0.061484 0.121775 0.18092 0.240256 0.300114 0.361146 0.423501 0.488669 0.553954 0.617581 0.680238 0.742187 0.804663 0.868259 0.93302 1 1 1 1 construction
  line L166 (11.4163, -14.103) -> (11.4042, -14.103) construction
  line L167 (11.4042, -14.103) -> (10.9657, -15.053) construction
  line L168 (10.9657, -15.053) -> (11.0584, -15.053) construction
  line L169 (11.0584, -15.053) -> (11.1988, -14.7485) construction
  line L170 (11.1988, -14.7485) -> (11.6295, -14.7485) construction
  line L171 (11.6295, -14.7485) -> (11.7739, -15.053) construction
  line L172 (11.7739, -15.053) -> (11.867, -15.053) construction
  line L173 (11.867, -15.053) -> (11.4163, -14.103) construction
  line L174 (12.4739, -15.053) -> (12.7683, -15.053) construction
  line L175 (12.7683, -15.053) -> (12.7683, -14.103) construction
  line L176 (12.7683, -14.103) -> (12.5764, -14.103) construction
  spline S24 degree 3 poles (12.5764, -14.103) (12.5598, -14.1031) (12.5275, -14.1034) (12.4809, -14.1048) (12.4378, -14.1074) (12.3984, -14.1112) (12.3624, -14.1159) (12.3301, -14.1217) (12.3012, -14.1286) (12.2834, -14.1345) (12.275, -14.1373) knots 0 0 0 0 0.164289 0.317406 0.458844 0.589367 0.707831 0.81577 0.91288 1 1 1 1 construction
  spline S25 degree 3 poles (12.275, -14.1373) (12.264, -14.1414) (12.2423, -14.1497) (12.2113, -14.1653) (12.1822, -14.183) (12.1547, -14.2028) (12.1295, -14.2253) (12.1057, -14.2495) (12.084, -14.2762) (12.0643, -14.305) (12.0464, -14.3355) (12.0309, -14.3676) (12.018, -14.4012) (12.0073, -14.4362) (11.9989, -14.4726) (11.9932, -14.5106) (11.9894, -14.5498) (11.989, -14.5765) (11.9888, -14.59) knots 0 0 0 0 0.061545 0.121694 0.181155 0.239875 0.298702 0.357647 0.417605 0.478494 0.540407 0.602345 0.665004 0.728559 0.793651 0.860534 0.929236 1 1 1 1 construction
  spline S26 degree 3 poles (11.9888, -14.59) (11.989, -14.6017) (11.9893, -14.6249) (11.9923, -14.659) (11.9967, -14.6921) (12.0035, -14.724) (12.0118, -14.755) (12.0223, -14.7848) (12.0344, -14.8137) (12.0486, -14.8412) (12.0641, -14.8673) (12.0807, -14.8919) (12.0985, -14.9146) (12.1175, -14.9356) (12.1376, -14.9547) (12.1589, -14.9722) (12.1814, -14.9878) (12.205, -15.0019) (12.2304, -15.0142) (12.2581, -15.0247) (12.2883, -15.0333) (12.3207, -15.0405) (12.3556, -15.0462) (12.3929, -15.0501) (12.4326, -15.0527) (12.4598, -15.0529) (12.4739, -15.053) knots 0 0 0 0 0.046081 0.090807 0.134295 0.177024 0.218823 0.260244 0.30108 0.341614 0.381583 0.42012 0.458075 0.494738 0.531195 0.566934 0.602713 0.638327 0.674853 0.713467 0.754442 0.797815 0.843989 0.893072 0.944963 1 1 1 1 construction
  spline S27 degree 3 poles (13.2345, -15.0774) (13.2417, -15.0772) (13.256, -15.0769) (13.277, -15.0745) (13.2977, -15.0711) (13.3177, -15.0656) (13.3372, -15.0589) (13.3563, -15.0508) (13.3748, -15.041) (13.393, -15.0297) (13.4106, -15.0167) (13.4277, -15.0015) (13.4448, -14.9846) (13.4612, -14.9655) (13.4775, -14.9445) (13.4932, -14.9214) (13.5087, -14.8964) (13.5184, -14.8788) (13.5234, -14.8697) knots 0 0 0 0 0.057208 0.113696 0.169178 0.224159 0.27872 0.333794 0.389241 0.445822 0.503704 0.564294 0.627975 0.695038 0.765373 0.839611 0.917538 1 1 1 1 construction
  line L177 (13.5234, -14.8697) -> (13.4431, -14.8216) construction
  spline S28 degree 3 poles (13.4431, -14.8216) (13.4356, -14.8341) (13.4213, -14.858) (13.3974, -14.8904) (13.3727, -14.9179) (13.3469, -14.9404) (13.3202, -14.9581) (13.2925, -14.9707) (13.2638, -14.9785) (13.2443, -14.9794) (13.2345, -14.9799) knots 0 0 0 0 0.159004 0.304646 0.438547 0.562322 0.677433 0.786897 0.893611 1 1 1 1 construction
  spline S29 degree 3 poles (13.2345, -14.9799) (13.2262, -14.9797) (13.2097, -14.9792) (13.1854, -14.9748) (13.1618, -14.968) (13.1393, -14.9583) (13.1184, -14.9465) (13.1001, -14.9323) (13.0842, -14.9164) (13.0712, -14.8987) (13.0613, -14.8796) (13.0536, -14.86) (13.0494, -14.8396) (13.0487, -14.8259) (13.0484, -14.8189) knots 0 0 0 0 0.091264 0.18093 0.270088 0.360156 0.448343 0.532666 0.613834 0.693982 0.772716 0.849335 0.923967 1 1 1 1 construction
  spline S30 degree 3 poles (13.0484, -14.8189) (13.0488, -14.811) (13.0496, -14.7949) (13.0565, -14.7712) (13.0673, -14.7477) (13.0773, -14.7332) (13.0825, -14.7257) knots 0 0 0 0 0.234723 0.477158 0.728556 1 1 1 1 construction
  spline S31 degree 3 poles (13.0825, -14.7257) (13.0867, -14.7202) (13.0956, -14.7088) (13.111, -14.6918) (13.129, -14.6743) (13.1491, -14.6555) (13.1719, -14.6364) (13.1968, -14.6161) (13.2244, -14.5953) (13.2438, -14.5814) (13.2537, -14.5742) knots 0 0 0 0 0.090279 0.18953 0.299198 0.418926 0.548376 0.688136 0.839084 1 1 1 1 construction
  spline S32 degree 3 poles (13.2537, -14.5742) (13.2637, -14.5671) (13.2828, -14.5535) (13.3096, -14.5333) (13.3335, -14.5148) (13.3544, -14.4979) (13.3725, -14.4825) (13.3877, -14.4689) (13.3997, -14.4566) (13.4064, -14.4486) (13.4094, -14.445) knots 0 0 0 0 0.181535 0.347082 0.495568 0.628357 0.74552 0.845831 0.930782 1 1 1 1 construction
  spline S33 degree 3 poles (13.4094, -14.445) (13.4136, -14.4394) (13.4219, -14.4284) (13.4328, -14.4112) (13.442, -14.3936) (13.4493, -14.3756) (13.4554, -14.3573) (13.4595, -14.3386) (13.4621, -14.3196) (13.4624, -14.3068) (13.4625, -14.3003) knots 0 0 0 0 0.133507 0.262559 0.388264 0.512667 0.633722 0.755394 0.877553 1 1 1 1 construction
  spline S34 degree 3 poles (13.4625, -14.3003) (13.4621, -14.2903) (13.4614, -14.2704) (13.4555, -14.2414) (13.4462, -14.2136) (13.4331, -14.1875) (13.4162, -14.1636) (13.3966, -14.1417) (13.3733, -14.1233) (13.3478, -14.1072) (13.3198, -14.0947) (13.2905, -14.0852) (13.2598, -14.0798) (13.239, -14.079) (13.2284, -14.0786) knots 0 0 0 0 0.083785 0.16578 0.24628 0.327461 0.408797 0.489715 0.571376 0.655523 0.741019 0.826547 0.911989 1 1 1 1 construction
  spline S35 degree 3 poles (13.2284, -14.0786) (13.2172, -14.079) (13.195, -14.0798) (13.1622, -14.0865) (13.1307, -14.0975) (13.1053, -14.1101) (13.0855, -14.1226) (13.0703, -14.134) (13.055, -14.1471) (13.0393, -14.162) (13.0236, -14.1788) (13.0076, -14.1974) (12.9912, -14.2176) (12.9807, -14.232) (12.9753, -14.2394) knots 0 0 0 0 0.107233 0.213252 0.31883 0.426794 0.483646 0.543604 0.608308 0.677127 0.750686 0.828713 0.91219 1 1 1 1 construction
  line L178 (12.9753, -14.2394) -> (13.0524, -14.2979) construction
  spline S36 degree 3 poles (13.0524, -14.2979) (13.0571, -14.2919) (13.066, -14.2803) (13.0796, -14.2642) (13.0924, -14.2494) (13.1051, -14.2366) (13.1169, -14.225) (13.1283, -14.215) (13.1392, -14.2067) (13.153, -14.1978) (13.1703, -14.1889) (13.192, -14.1815) (13.2147, -14.177) (13.2301, -14.1764) (13.2379, -14.1761) knots 0 0 0 0 0.098469 0.189629 0.274184 0.352183 0.423199 0.488551 0.548473 0.60144 0.701198 0.799592 0.898545 1 1 1 1 construction
  spline S37 degree 3 poles (13.2379, -14.1761) (13.2478, -14.1764) (13.2667, -14.177) (13.2936, -14.184) (13.3177, -14.1949) (13.3385, -14.2102) (13.3558, -14.2283) (13.3683, -14.2491) (13.3759, -14.2721) (13.3768, -14.2882) (13.3772, -14.2963) knots 0 0 0 0 0.143073 0.275903 0.402371 0.528414 0.650356 0.765895 0.880774 1 1 1 1 construction
  spline S38 degree 3 poles (13.3772, -14.2963) (13.3771, -14.3014) (13.3769, -14.3116) (13.3739, -14.3267) (13.3701, -14.3417) (13.3641, -14.3566) (13.3557, -14.3717) (13.3447, -14.3871) (13.3308, -14.4032) (13.3202, -14.4136) (13.3146, -14.4191) knots 0 0 0 0 0.107285 0.214746 0.322939 0.434116 0.553412 0.686073 0.834256 1 1 1 1 construction
  spline S39 degree 3 poles (13.3146, -14.4191) (13.3126, -14.421) (13.3076, -14.4254) (13.2986, -14.4326) (13.2867, -14.4415) (13.2721, -14.4525) (13.2548, -14.4653) (13.2346, -14.4797) (13.2117, -14.4961) (13.1955, -14.5076) (13.1869, -14.5137) knots 0 0 0 0 0.052594 0.124952 0.218094 0.333502 0.468789 0.624938 0.801683 1 1 1 1 construction
  spline S40 degree 3 poles (13.1869, -14.5137) (13.1766, -14.5212) (13.1567, -14.5357) (13.1283, -14.5575) (13.1025, -14.5789) (13.0793, -14.5996) (13.0584, -14.6196) (13.0401, -14.639) (13.0242, -14.6577) (13.0071, -14.6818) (12.9895, -14.7113) (12.9745, -14.7475) (12.965, -14.7838) (12.9638, -14.8082) (12.9631, -14.8203) knots 0 0 0 0 0.096972 0.187773 0.272396 0.351321 0.424335 0.491909 0.554233 0.611268 0.716348 0.81454 0.908495 1 1 1 1 construction
  spline S41 degree 3 poles (12.9631, -14.8203) (12.9633, -14.8288) (12.9637, -14.8456) (12.9677, -14.8704) (12.9737, -14.8945) (12.9827, -14.9175) (12.9936, -14.94) (13.0075, -14.9613) (13.0236, -14.9818) (13.0421, -15.0012) (13.0623, -15.0189) (13.0836, -15.0347) (13.1062, -15.0478) (13.1298, -15.0586) (13.1544, -15.067) (13.1802, -15.073) (13.207, -15.0768) (13.2252, -15.0772) (13.2345, -15.0774) knots 0 0 0 0 0.061484 0.121775 0.18092 0.240256 0.300114 0.361146 0.423501 0.488669 0.553954 0.617581 0.680238 0.742187 0.804663 0.868259 0.93302 1 1 1 1 construction
  spline S42 degree 3 poles (10.9783, -11.4953) (10.9674, -11.4954) (10.9457, -11.4957) (10.9138, -11.4982) (10.8827, -11.5024) (10.8524, -11.5082) (10.8228, -11.5153) (10.794, -11.5245) (10.7661, -11.5351) (10.739, -11.5473) (10.7129, -11.561) (10.688, -11.5761) (10.6642, -11.5924) (10.6416, -11.61) (10.6204, -11.6291) (10.6, -11.6492) (10.5812, -11.671) (10.5696, -11.6863) (10.5638, -11.694) knots 0 0 0 0 0.068548 0.135683 0.201215 0.265682 0.329267 0.392395 0.45507 0.517127 0.57879 0.63974 0.700192 0.759806 0.819628 0.879355 0.939512 1 1 1 1 construction
  line L179 (10.5638, -11.694) -> (10.6384, -11.7511) construction
  spline S43 degree 3 poles (10.6384, -11.7511) (10.6437, -11.7447) (10.6543, -11.7321) (10.6713, -11.7144) (10.689, -11.6979) (10.7074, -11.6823) (10.7269, -11.6684) (10.747, -11.6553) (10.7679, -11.6435) (10.7969, -11.6293) (10.8348, -11.6144) (10.8825, -11.602) (10.9323, -11.594) (10.9663, -11.5932) (10.9836, -11.5927) knots 0 0 0 0 0.063163 0.125475 0.187121 0.248294 0.309295 0.36985 0.430973 0.492456 0.616148 0.740844 0.868183 1 1 1 1 construction
  spline S44 degree 3 poles (10.9836, -11.5927) (10.9931, -11.5929) (11.0121, -11.5931) (11.0402, -11.596) (11.0678, -11.6) (11.0949, -11.606) (11.1214, -11.6136) (11.1475, -11.6227) (11.1728, -11.6339) (11.1976, -11.6463) (11.2214, -11.6603) (11.244, -11.6756) (11.2652, -11.692) (11.285, -11.7095) (11.3035, -11.7282) (11.3205, -11.7481) (11.3361, -11.7692) (11.3504, -11.7913) (11.3632, -11.8142) (11.3739, -11.8381) (11.3834, -11.8626) (11.3909, -11.8879) (11.3969, -11.9138) (11.401, -11.9405) (11.4038, -11.9678) (11.4041, -11.9863) (11.4042, -11.9956) knots 0 0 0 0 0.043955 0.087502 0.130463 0.172752 0.215403 0.25765 0.300153 0.343121 0.385925 0.427686 0.468818 0.509492 0.549883 0.58998 0.630405 0.670869 0.711384 0.751627 0.791776 0.832459 0.873319 0.914543 0.956924 1 1 1 1 construction
  spline S45 degree 3 poles (11.4042, -11.9956) (11.4038, -12.0097) (11.4032, -12.0372) (11.3972, -12.0776) (11.3881, -12.1163) (11.3744, -12.153) (11.3576, -12.1883) (11.3364, -12.2215) (11.3118, -12.2531) (11.2835, -12.2823) (11.2525, -12.3091) (11.2191, -12.3326) (11.1836, -12.3523) (11.1463, -12.3686) (11.107, -12.3812) (11.0656, -12.39) (11.0223, -12.3958) (10.9928, -12.3963) (10.9777, -12.3966) knots 0 0 0 0 0.064323 0.12629 0.186726 0.246146 0.305576 0.365429 0.426326 0.48884 0.551725 0.613919 0.675484 0.737334 0.800229 0.864502 0.931041 1 1 1 1 construction
  spline S46 degree 3 poles (10.9777, -12.3966) (10.9611, -12.3961) (10.9285, -12.3952) (10.8806, -12.3876) (10.8348, -12.3752) (10.791, -12.3578) (10.7494, -12.3353) (10.7098, -12.308) (10.6724, -12.2756) (10.6499, -12.2509) (10.6384, -12.2383) knots 0 0 0 0 0.128515 0.252949 0.374755 0.49594 0.617181 0.740909 0.867811 1 1 1 1 construction
  line L180 (10.6384, -12.2383) -> (10.5638, -12.2948) construction
  spline S47 degree 3 poles (10.5638, -12.2948) (10.5698, -12.3025) (10.5818, -12.318) (10.6012, -12.3398) (10.6216, -12.3603) (10.6432, -12.3793) (10.6658, -12.3973) (10.6897, -12.4136) (10.7146, -12.4286) (10.7405, -12.4424) (10.7673, -12.4546) (10.795, -12.465) (10.8234, -12.474) (10.8527, -12.4814) (10.8827, -12.4872) (10.9135, -12.491) (10.945, -12.4937) (10.9663, -12.4939) (10.9771, -12.494) knots 0 0 0 0 0.061674 0.123053 0.183475 0.243727 0.304279 0.364863 0.425946 0.487391 0.54922 0.611144 0.673529 0.736961 0.800785 0.866013 0.932101 1 1 1 1 construction
  spline S48 degree 3 poles (10.9771, -12.494) (10.9873, -12.494) (11.0075, -12.4938) (11.0374, -12.4915) (11.0664, -12.4884) (11.0946, -12.4837) (11.122, -12.4782) (11.1485, -12.4708) (11.1743, -12.4625) (11.1993, -12.4528) (11.2234, -12.4418) (11.2467, -12.4294) (11.2692, -12.4156) (11.2909, -12.4008) (11.3117, -12.3845) (11.3317, -12.367) (11.351, -12.3482) (11.363, -12.3347) (11.369, -12.3279) knots 0 0 0 0 0.069663 0.13775 0.203917 0.26878 0.332414 0.394754 0.45618 0.516996 0.577396 0.637198 0.696999 0.756756 0.816554 0.876948 0.938132 1 1 1 1 construction
  spline S49 degree 3 poles (11.369, -12.3279) (11.3786, -12.3161) (11.3977, -12.2926) (11.4222, -12.2545) (11.4431, -12.2147) (11.46, -12.1731) (11.4733, -12.1297) (11.4824, -12.0844) (11.4884, -12.0374) (11.4891, -12.0054) (11.4894, -11.9891) knots 0 0 0 0 0.124329 0.247156 0.36878 0.490734 0.613614 0.738958 0.867311 1 1 1 1 construction
  spline S50 degree 3 poles (11.4894, -11.9891) (11.489, -11.9721) (11.4882, -11.9384) (11.4811, -11.8891) (11.4698, -11.8418) (11.4536, -11.7967) (11.4332, -11.7535) (11.408, -11.7126) (11.3782, -11.6736) (11.3441, -11.6373) (11.3068, -11.604) (11.2668, -11.5747) (11.2243, -11.5504) (11.1796, -11.53) (11.1325, -11.5144) (11.0831, -11.5034) (11.0314, -11.4966) (10.9962, -11.4957) (10.9783, -11.4953) knots 0 0 0 0 0.064558 0.127014 0.187955 0.248014 0.307748 0.368235 0.42947 0.492743 0.556258 0.618217 0.679655 0.741246 0.803415 0.866815 0.932328 1 1 1 1 construction
  spline S51 degree 3 poles (12.0501, -11.4953) (12.0391, -11.4954) (12.0175, -11.4957) (11.9856, -11.4982) (11.9545, -11.5024) (11.9242, -11.5082) (11.8946, -11.5153) (11.8658, -11.5245) (11.8378, -11.5351) (11.8108, -11.5473) (11.7847, -11.561) (11.7598, -11.5761) (11.736, -11.5924) (11.7134, -11.61) (11.6921, -11.6291) (11.6718, -11.6492) (11.653, -11.671) (11.6414, -11.6863) (11.6356, -11.694) knots 0 0 0 0 0.068548 0.135683 0.201215 0.265682 0.329267 0.392395 0.45507 0.517127 0.57879 0.63974 0.700192 0.759806 0.819628 0.879355 0.939512 1 1 1 1 construction
  line L181 (11.6356, -11.694) -> (11.7102, -11.7511) construction
  spline S52 degree 3 poles (11.7102, -11.7511) (11.7155, -11.7447) (11.7261, -11.7321) (11.7431, -11.7144) (11.7608, -11.6979) (11.7792, -11.6823) (11.7987, -11.6684) (11.8188, -11.6553) (11.8397, -11.6435) (11.8687, -11.6293) (11.9066, -11.6144) (11.9543, -11.602) (12.0041, -11.594) (12.0381, -11.5932) (12.0554, -11.5927) knots 0 0 0 0 0.063163 0.125475 0.187121 0.248294 0.309295 0.36985 0.430973 0.492456 0.616148 0.740844 0.868183 1 1 1 1 construction
  spline S53 degree 3 poles (12.0554, -11.5927) (12.0649, -11.5929) (12.0839, -11.5931) (12.112, -11.596) (12.1396, -11.6) (12.1667, -11.606) (12.1932, -11.6136) (12.2192, -11.6227) (12.2445, -11.6339) (12.2694, -11.6463) (12.2932, -11.6603) (12.3158, -11.6756) (12.337, -11.692) (12.3568, -11.7095) (12.3753, -11.7282) (12.3923, -11.7481) (12.4079, -11.7692) (12.4222, -11.7913) (12.435, -11.8142) (12.4457, -11.8381) (12.4552, -11.8626) (12.4627, -11.8879) (12.4687, -11.9138) (12.4728, -11.9405) (12.4756, -11.9678) (12.4759, -11.9863) (12.476, -11.9956) knots 0 0 0 0 0.043955 0.087502 0.130463 0.172752 0.215403 0.25765 0.300153 0.343121 0.385925 0.427686 0.468818 0.509492 0.549883 0.58998 0.630405 0.670869 0.711384 0.751627 0.791776 0.832459 0.873319 0.914543 0.956924 1 1 1 1 construction
  spline S54 degree 3 poles (12.476, -11.9956) (12.4756, -12.0097) (12.4749, -12.0372) (12.469, -12.0776) (12.4599, -12.1163) (12.4462, -12.153) (12.4294, -12.1883) (12.4082, -12.2215) (12.3836, -12.2531) (12.3553, -12.2823) (12.3242, -12.3091) (12.2909, -12.3326) (12.2554, -12.3523) (12.2181, -12.3686) (12.1788, -12.3812) (12.1374, -12.39) (12.0941, -12.3958) (12.0645, -12.3963) (12.0495, -12.3966) knots 0 0 0 0 0.064323 0.12629 0.186726 0.246146 0.305576 0.365429 0.426326 0.48884 0.551725 0.613919 0.675484 0.737334 0.800229 0.864502 0.931041 1 1 1 1 construction
  spline S55 degree 3 poles (12.0495, -12.3966) (12.0329, -12.3961) (12.0003, -12.3952) (11.9524, -12.3876) (11.9066, -12.3752) (11.8628, -12.3578) (11.8212, -12.3353) (11.7816, -12.308) (11.7442, -12.2756) (11.7217, -12.2509) (11.7102, -12.2383) knots 0 0 0 0 0.128515 0.252949 0.374755 0.49594 0.617181 0.740909 0.867811 1 1 1 1 construction
  line L182 (11.7102, -12.2383) -> (11.6356, -12.2948) construction
  spline S56 degree 3 poles (11.6356, -12.2948) (11.6416, -12.3025) (11.6536, -12.318) (11.673, -12.3398) (11.6934, -12.3603) (11.715, -12.3793) (11.7376, -12.3973) (11.7615, -12.4136) (11.7864, -12.4286) (11.8123, -12.4424) (11.8391, -12.4546) (11.8668, -12.465) (11.8952, -12.474) (11.9245, -12.4814) (11.9545, -12.4872) (11.9853, -12.491) (12.0168, -12.4937) (12.0381, -12.4939) (12.0489, -12.494) knots 0 0 0 0 0.061674 0.123053 0.183475 0.243727 0.304279 0.364863 0.425946 0.487391 0.54922 0.611144 0.673529 0.736961 0.800785 0.866013 0.932101 1 1 1 1 construction
  spline S57 degree 3 poles (12.0489, -12.494) (12.0591, -12.494) (12.0793, -12.4938) (12.1092, -12.4915) (12.1382, -12.4884) (12.1664, -12.4837) (12.1938, -12.4782) (12.2203, -12.4708) (12.2461, -12.4625) (12.271, -12.4528) (12.2952, -12.4418) (12.3185, -12.4294) (12.341, -12.4156) (12.3627, -12.4008) (12.3835, -12.3845) (12.4035, -12.367) (12.4228, -12.3482) (12.4348, -12.3347) (12.4408, -12.3279) knots 0 0 0 0 0.069663 0.13775 0.203917 0.26878 0.332414 0.394754 0.45618 0.516996 0.577396 0.637198 0.696999 0.756756 0.816554 0.876948 0.938132 1 1 1 1 construction
  spline S58 degree 3 poles (12.4408, -12.3279) (12.4504, -12.3161) (12.4695, -12.2926) (12.494, -12.2545) (12.5149, -12.2147) (12.5318, -12.1731) (12.5451, -12.1297) (12.5542, -12.0844) (12.5602, -12.0374) (12.5609, -12.0054) (12.5612, -11.9891) knots 0 0 0 0 0.124329 0.247156 0.36878 0.490734 0.613614 0.738958 0.867311 1 1 1 1 construction
  spline S59 degree 3 poles (12.5612, -11.9891) (12.5608, -11.9721) (12.56, -11.9384) (12.5529, -11.8891) (12.5416, -11.8418) (12.5254, -11.7967) (12.505, -11.7535) (12.4797, -11.7126) (12.45, -11.6736) (12.4159, -11.6373) (12.3786, -11.604) (12.3386, -11.5747) (12.2961, -11.5504) (12.2514, -11.53) (12.2043, -11.5144) (12.1549, -11.5034) (12.1032, -11.4966) (12.068, -11.4957) (12.0501, -11.4953) knots 0 0 0 0 0.064558 0.127014 0.187955 0.248014 0.307748 0.368235 0.42947 0.492743 0.556258 0.618217 0.679655 0.741246 0.803415 0.866815 0.932328 1 1 1 1 construction
  line L183 (13.0971, -12.4697) -> (13.499, -11.5197) construction
  line L184 (13.499, -11.5197) -> (13.4077, -11.5197) construction
  line L185 (13.4077, -11.5197) -> (13.091, -12.2683) construction
  line L186 (13.091, -12.2683) -> (12.7744, -11.5197) construction
  line L187 (12.7744, -11.5197) -> (12.683, -11.5197) construction
  line L188 (12.683, -11.5197) -> (13.0849, -12.4697) construction
  line L189 (13.0849, -12.4697) -> (13.0971, -12.4697) construction
  line L190 (11.0123, -9.8863) -> (11.3067, -9.8863) construction
  line L191 (11.3067, -9.8863) -> (11.3067, -8.9363) construction
  line L192 (11.3067, -8.9363) -> (11.1149, -8.9363) construction
  spline S60 degree 3 poles (11.1149, -8.9363) (11.0982, -8.9365) (11.066, -8.9367) (11.0194, -8.9382) (10.9763, -8.9408) (10.9368, -8.9446) (10.9009, -8.9492) (10.8685, -8.955) (10.8396, -8.9619) (10.8219, -8.9678) (10.8135, -8.9706) knots 0 0 0 0 0.164289 0.317406 0.458844 0.589367 0.707831 0.81577 0.91288 1 1 1 1 construction
  spline S61 degree 3 poles (10.8135, -8.9706) (10.8025, -8.9748) (10.7807, -8.9831) (10.7498, -8.9987) (10.7207, -9.0164) (10.6932, -9.0362) (10.668, -9.0586) (10.6441, -9.0828) (10.6225, -9.1096) (10.6027, -9.1384) (10.5849, -9.1689) (10.5694, -9.201) (10.5565, -9.2346) (10.5458, -9.2695) (10.5374, -9.306) (10.5316, -9.3439) (10.5278, -9.3832) (10.5274, -9.4098) (10.5272, -9.4233) knots 0 0 0 0 0.061545 0.121694 0.181155 0.239875 0.298702 0.357647 0.417605 0.478494 0.540407 0.602345 0.665004 0.728559 0.793651 0.860534 0.929236 1 1 1 1 construction
  spline S62 degree 3 poles (10.5272, -9.4233) (10.5274, -9.4351) (10.5278, -9.4582) (10.5308, -9.4923) (10.5352, -9.5254) (10.542, -9.5573) (10.5502, -9.5884) (10.5608, -9.6182) (10.5729, -9.647) (10.587, -9.6746) (10.6025, -9.7006) (10.6192, -9.7252) (10.637, -9.748) (10.656, -9.7689) (10.6761, -9.7881) (10.6973, -9.8056) (10.7198, -9.8211) (10.7434, -9.8352) (10.7689, -9.8476) (10.7966, -9.858) (10.8267, -9.8666) (10.8592, -9.8738) (10.8941, -9.8796) (10.9314, -9.8834) (10.9711, -9.886) (10.9983, -9.8862) (11.0123, -9.8863) knots 0 0 0 0 0.046081 0.090807 0.134295 0.177024 0.218823 0.260244 0.30108 0.341614 0.381583 0.42012 0.458075 0.494738 0.531195 0.566934 0.602713 0.638327 0.674853 0.713467 0.754442 0.797815 0.843989 0.893072 0.944963 1 1 1 1 construction
  line L193 (12.1958, -9.8863) -> (12.2811, -9.8863) construction
  line L194 (12.2811, -9.8863) -> (12.2811, -8.9363) construction
  line L195 (12.2811, -8.9363) -> (12.2632, -8.9363) construction
  line L196 (12.2632, -8.9363) -> (11.6356, -9.684) construction